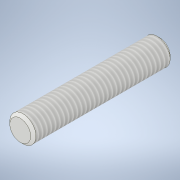
# Autodesk Inventor part: Dowel Pin
Saved by Autodesk Inventor 2022 (Build 260153000, 153)
## iProperties
Created: 2021-10-05
Part Number: Dowel Pin
Material: Generic
Document SubType Name: Modeling
Designer: Administrator
Density: 1 g/cm^3
Appearance: Default
Mass: 0.14058 g
Surface Area: 1.99086 cm^2
Volume: 0.14058 cm^3
Title: Dowel Pin v2
Author: Administrator
Autodesk Inventor part; units mm, degrees
ref_plane "YZ Plane" through (0, 0, 0) normal (1, 0, 0) x (0, 1, 0)
ref_plane "XZ Plane" through (0, 0, 0) normal (0, 1, 0) x (-1, 0, 0)
ref_plane "XY Plane" through (0, 0, 0) normal (0, 0, 1) x (1, 0, 0)
sketch "Sketch1" plane through (0, 0, 0) normal (0, 0, 1) x (1, 0, 0)
  circle A0 centre (0, 0) radius 1.5
  constraints: 1 centre point
extrude "Extrusion1" add sketch "Sketch1" along normal blind 16
chamfer "Chamfer2" distance 0.3 angle 45 1 edges at (-1.5, 0, 16)
chamfer "Chamfer1" distance 0.3 angle 45 1 edges at (-1.5, 0, 0)
thread "Thread1" size "M3x0.5" class "6g" standard "ANSI Metric M Profile" full length
sketch "Sketch2" plane through (0, 0, 0) normal (0, 0, -1) x (-1, 0, 0)
  line L0 (-0.75, -0.433) -> (-0.75, 0.433)
  line L1 (-0.75, 0.433) -> (0, 0.866)
  line L2 (0, 0.866) -> (0.75, 0.433)
  line L3 (0.75, 0.433) -> (0.75, -0.433)
  line L4 (0.75, -0.433) -> (0, -0.866)
  line L5 (0, -0.866) -> (-0.75, -0.433)
  point P0 (0, 0)
  point P1 (0, 0)
  dimension "d10" = 1.5
  constraints: 12 end point, 1 coincident, 1 vertical, 13 other
  measures "d10" distance between parallel lines of L3 L0
extrude "Extrusion2" cut sketch "Sketch2" against normal blind 2
body "Solid3"
